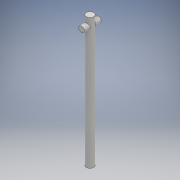
# Autodesk Inventor part: Handle
Saved by Autodesk Inventor 2018 (Build 220112000, 112)
## iProperties
Created: 2019-07-18
Part Number: Handle
Material: Generic
Document SubType Name: Modeling
Designer: aal_9
Density: 1 g/cm^3
Appearance: Default
Author: aal_9
Autodesk Inventor part; units mm, degrees
ref_plane "YZ Plane" through (0, 0, 0) normal (1, 0, 0) x (0, 1, 0)
ref_plane "XY Plane" through (0, 0, 0) normal (0, 0, 1) x (1, 0, 0)
sketch "Sketch1" plane through (0, 0, 0) normal (0, 0, 1) x (1, 0, 0)
  circle A0 centre (0, 0) radius 3.2
  dimension "d0" = 6.4
  constraints: 1 centre point, 1 coincident
  measures "d0" diameter of A0
extrude "Extrusion1" add sketch "Sketch1" along normal blind 115
ref_plane "Work Plane1" through (0, 3.2, 0) normal (0, 1, 0) x (-1, 0, 0)
sketch "Sketch2" plane through (0, 3.2, 0) normal (0, 1, 0) x (-1, 0, 0)
  line L0 (0, -23) -> (0, 138) projected
  circle A0 centre (0, 107.5) radius 2.5
  line L1 (3.2, 115) -> (-3.2, 115) projected
  point P0 (0, 0)
  dimension "d11" = 5
  dimension "d12" = 7.5
  constraints: 1 centre point, 1 point on line
  measures "d11" diameter of A0
  measures "d12" distance from line of L1 A0.centre
extrude "Extrusion2" add sketch "Sketch2" along normal blind 4.25 and the other way blind 10.65
body "Solid1"
